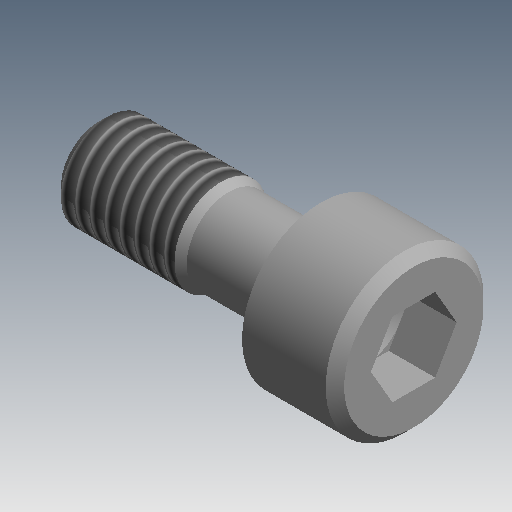
# Autodesk Inventor part: HCBST5-12_s
Saved by Autodesk Inventor 2020 (Build 240168000, 168)
## iProperties
Part Number: HCBST5-12_s
Material: Generic
Catalog Web Link: www.cadenas.de
Description: HCBST_secscrew-Frame Washer Assembled Hexagon Socket Head Cap Screws for Aluminum Frames
Vendor: MISUMI
Document SubType Name: Modeling
Designer: partserver
Manufacturer: MISUMI
Mass: 0.455842 g
Surface Area: 4.5576 cm^2
Volume: 0.455842 cm^3
Density: 1 g/cm^3
Appearance: PSOLRGB-192-192-192
Category: PARTsolutions
Company: MISUMI
PSOL_IDENT_0: {$CADENAS_DATA\23d-libs\misumi\metric\38_al_extrusions_blackets\38_accessories\sec_parts\sec_screw.p
PSOL_IDENT_1: rj},170 {VTYP=3D},{NB=HCBST5-12_s},{LINA=HCBST5-12},{NN=HCBST_secscrew},{DATE=30.03.2018 06:53:28},{
PSOL_IDENT_2: GEOMDATE=13.10.2015 01:08:00},{VERSION=},{LINEID=40},{WBVAR=L},{WBNUMERIC=L}  {NB=HCBST5-12_s},{LINA=
PSOL_IDENT_3: HCBST5-12},{KT=DUMMY},{PN=HCBST5-12},{TYPE=HCBST},{M=5},{L=12},{M1=5.000},{L0=12},{NDM=5},{KDM=4.017
PSOL_IDENT_4: 064},{MP=5X0.8},{P=0.8},{A=8.5},{E=5},{B=4},{C=9.2},{D=10.0},{AA=5.4},{TT1=1.3},{TT2=1},{DDC=5.1},{D
PSOL_IDENT_5: DD=5.3}
NB: HCBST5-12_s
NN: HCBST_secscrew
NT: Frame Washer Assembled Hexagon Socket Head Cap Screws for Aluminum Frames
NBSYN: $PN._s
LINA: HCBST5-12
CATALOG: Misumi
PN: HCBST5-12
M: 5
L: 12
MP: 5X0.8
A: 8.5
E: 5
B: 4
C: 9.2
D: 10
SUPPLIER: MISUMI
ARTICLENO: HCBST5-12_s
BOMINFO: HCBST5-12
CREATOR: CADENAS GmbH
Title: HCBST5-12
Author: Cadenas PARTsolutions
Comments: Frame Washer Assembled Hexagon Socket Head Cap Screws for Aluminum Frames
Autodesk Inventor part; units mm, degrees
sketch "Sketch_6" plane through (0, 0, 0) normal (0, 0, 1) x (1, 0, 0)
  line L0 (12, 0) -> (4.5504, 0)
  line L1 (4.5504, 0) -> (4.5504, 2.0095)
  line L2 (4.5504, 2.0095) -> (5.4, 2.5)
  line L3 (5.4, 2.5) -> (11.5095, 2.5)
  line L4 (11.5095, 2.5) -> (12, 2.0095)
  line L5 (12, 2.0095) -> (12, 0)
  line L6 (12, 0) -> (4.5504, 0)
  constraints: 14 end point
revolve "Revolution1" add sketch "Sketch_6" angle 360 about axis through (12, 0, 0) along (1, 0, 0)
thread "Thread1" size "M5x0.8" class "6g" standard "ISO Metric profile" full length
sketch "Sketch_1" plane through (0, 0, 0) normal (0, 0, 1) x (1, 0, 0)
  line L0 (5.4, 0) -> (-5, 0)
  line L1 (-1.3453, 0) -> (-2.5, 2)
  line L2 (-2.5, 2) -> (-5, 2)
  line L3 (-5, 2) -> (-5, 3.75)
  line L4 (-5, 3.75) -> (-4.5, 4.25)
  line L5 (-4.5, 4.25) -> (0, 4.25)
  line L6 (0, 4.25) -> (0, 2.2543)
  line L7 (0, 2.2543) -> (5.4, 2.2543)
  line L8 (5.4, 2.2543) -> (5.4, 0)
  line L9 (5.4, 0) -> (-1.3453, 0)
  constraints: 20 end point
revolve "Revolution2" add sketch "Sketch_1" angle 360 about axis through (5.4, 0, 0) along (1, 0, 0)
sketch "Sketch_2" plane through (-5, 0, 0) normal (1, 0, 0) x (0, 0, -1)
  line L0 (-2, -1.1547) -> (0, -2.3094)
  line L1 (0, -2.3094) -> (2, -1.1547)
  line L2 (2, -1.1547) -> (2, 1.1547)
  line L3 (2, 1.1547) -> (0, 2.3094)
  line L4 (0, 2.3094) -> (-2, 1.1547)
  line L5 (-2, 1.1547) -> (-2, -1.1547)
  constraints: 12 end point
extrude "Extrusion1" cut sketch "Sketch_2" along normal blind 2.5
ref_plane "bolt_to_plane_washer_XY" through (1.3, 0, 0) normal (1, 0, 0) x (0, 0, -1)
ref_plane "bolt_to_plane_washer_YZ" through (1.3, 0, 0) normal (0, 0, -1) x (0, 1, 0)
ref_plane "bolt_to_plane_washer_ZX" through (1.3, 0, 0) normal (0, 1, 0) x (1, 0, 0)
ref_plane "bolt_to_spring_washer_XY" through (0, 0, 0) normal (1, 0, 0) x (0, 0, -1)
ref_plane "bolt_to_spring_washer_YZ" through (0, 0, 0) normal (0, 0, -1) x (0, 1, 0)
ref_plane "bolt_to_spring_washer_ZX" through (0, 0, 0) normal (0, 1, 0) x (1, 0, 0)
ref_plane "to_body_XY" through (2.3, 0, 0) normal (1, 0, 0) x (0, 0, -1)
ref_plane "to_body_YZ" through (2.3, 0, 0) normal (0, 0, -1) x (0, 1, 0)
ref_plane "to_body_ZX" through (2.3, 0, 0) normal (0, 1, 0) x (1, 0, 0)
ref_plane "to_nut_XY" through (12, 0, 0) normal (1, 0, 0) x (0, 0, -1)
ref_plane "to_nut_YZ" through (12, 0, 0) normal (0, 0, -1) x (0, 1, 0)
ref_plane "to_nut_ZX" through (12, 0, 0) normal (0, 1, 0) x (1, 0, 0)
body "Solid1"
